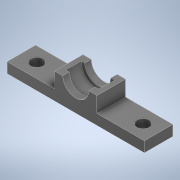
# Autodesk Inventor part: Mancal inferior
Saved by Autodesk Inventor 2021 (Build 250183000, 183)
## iProperties
Created: 2021-11-16
Part Number: Mancal inferior
Material: Generic
Document SubType Name: Modeling
Designer: Mathe
Density: 1 g/cm^3
Appearance: Smooth - Black
Author: Mathe
Autodesk Inventor part; units mm, degrees
ref_plane "YZ Plane" through (0, 0, 0) normal (1, 0, 0) x (0, 1, 0)
ref_plane "XZ Plane" through (0, 0, 0) normal (0, 1, 0) x (-1, 0, 0)
ref_plane "XY Plane" through (0, 0, 0) normal (0, 0, 1) x (1, 0, 0)
sketch "Sketch1" plane through (0, 0, 0) normal (0, 0, 1) x (1, 0, 0)
  line L0 (0, 6) -> (0, -1) construction
  line L1 (-13.25, 0) -> (13.25, 0)
  line L2 (13.25, 0) -> (13.25, 2)
  line L3 (-13.25, 0) -> (-13.25, 2)
  line L4 (-13.25, 2) -> (-4.1, 2)
  line L5 (-4.1, 2) -> (-4.1, 5)
  line L6 (-4.1, 5) -> (-2.5, 5)
  line L7 (13.25, 2) -> (4.1, 2)
  line L8 (4.1, 2) -> (4.1, 5)
  line L9 (4.1, 5) -> (2.5, 5)
  arc A0 (-2.5, 5) -> (2.5, 5) centre (0, 5) ccw
  line L10 (-18.55, 0) -> (18.55, 0) construction
  point P0 (0, 0)
  dimension "d0" = 2
  dimension "d1" = 2.5
  dimension "d2" = 8.2
  dimension "d3" = 26.5
  dimension "d6" = 3
  constraints: 18 end point, 4 perpendicular, 3 collinear, 3 vertical, 2 horizontal, 2 point on circle, 2 point on line, 1 centre point, 2 other
  measures "d0" distance of L1.end L2.end
  measures "d1" radius of A0
  measures "d2" distance between parallel lines of L8 L5
  measures "d3" distance of L1.start L1.end
  measures "d6" distance of L7.end L8.end
extrude "Extrusion1" add sketch "Sketch1" along normal mid plane 5.5
sketch "Sketch2" plane through (0, 0, 0) normal (0, 0, 1) x (1, 0, 0)
  arc A0 (-2.5, 5) -> (2.5, 5) centre (0, 5) ccw construction
  arc A1 (-3.2, 5) -> (3.2, 5) centre (0, 5) ccw
  line L0 (-3.2, 5) -> (3.2, 5)
  line L1 (4.1, 5) -> (2.5, 5) construction
  line L2 (-2.5, 5) -> (-4.1, 5) construction
  point P0 (0, 0)
  dimension "d9" = 6.4
  constraints: 2 end point, 2 point on circle, 2 point on line, 1 centre point, 1 coincident, 1 collinear
  measures "d9" diameter of A1
extrude "Extrusion2" cut sketch "Sketch2" along normal mid plane 3
sketch "Sketch3" plane through (-13.25, 2, 2.75) normal (0, 1, 0) x (1, 0, 0)
  line L0 (-5.3, 2.75) -> (31.8, 2.75) construction
  line L1 (13.25, 6.6) -> (13.25, -1.1) construction
  circle A0 centre (3, 2.75) radius 1.2
  circle A1 centre (23.5, 2.75) radius 1.2
  line L2 (0, 5.5) -> (0, 0) construction
  point P0 (13.25, 2.75)
  dimension "d12" = 3
  dimension "d13" = 2.4
  constraints: 2 centre point, 2 point on line, 1 equal radius, 1 symmetric about line
  measures "d12" distance from line of L2 A0.centre
  measures "d13" diameter of A0
extrude "Extrusion3" cut sketch "Sketch3" against normal up to surface (2 mm away)
body "Solid1"
